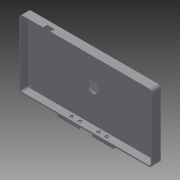
# Autodesk Inventor part: Master Tablet Enclosure
Saved by Autodesk Inventor 2014 SP2 (Build 180246200, 246)
## iProperties
Created: 2015-08-04
Part Number: Master Tablet Enclosure
Material: Generic
Document SubType Name: Modeling
Designer: Devon
Density: 1 g/cm^3
Appearance: Default
Author: Devon
Autodesk Inventor part; units mm, degrees
ref_plane "YZ Plane" through (0, 0, 0) normal (1, 0, 0) x (0, 1, 0)
ref_plane "XZ Plane" through (0, 0, 0) normal (0, 1, 0) x (-1, 0, 0)
sketch "Sketch1" plane through (0, 0, 0) normal (0, 0, 1) x (1, 0, 0)
  line L0 (-10.454202, 14.601943) -> (210.208298, 14.601943)
  line L1 (216.558298, 8.251943) -> (216.558298, -98.110557)
  line L2 (210.208298, -104.460557) -> (-10.454202, -104.460557)
  line L3 (-16.804202, -98.110557) -> (-16.804202, 8.251943)
  line L4 (99.877048, 12.220693) -> (-10.454202, 12.220693)
  line L5 (-14.422952, 8.251943) -> (-14.422952, -44.929307)
  line L6 (99.877048, 12.220693) -> (210.208298, 12.220693)
  line L7 (214.177048, 8.251943) -> (214.177048, -44.929307)
  line L8 (99.877048, -102.079307) -> (210.208298, -102.079307)
  line L9 (214.177048, -98.110557) -> (214.177048, -44.929307)
  line L10 (99.877048, -102.079307) -> (-10.454202, -102.079307)
  line L11 (-14.422952, -98.110557) -> (-14.422952, -44.929307)
  arc A0 (-10.454202, 14.601943) -> (-16.804202, 8.251943) centre (-10.454202, 8.251943) ccw
  arc A1 (216.558298, 8.251943) -> (210.208298, 14.601943) centre (210.208298, 8.251943) ccw
  arc A2 (210.208298, -104.460557) -> (216.558298, -98.110557) centre (210.208298, -98.110557) ccw
  arc A3 (-16.804202, -98.110557) -> (-10.454202, -104.460557) centre (-10.454202, -98.110557) ccw
  arc A4 (-10.454202, 12.220693) -> (-14.422952, 8.251943) centre (-10.454202, 8.251943) ccw
  arc A5 (214.177048, 8.251943) -> (210.208298, 12.220693) centre (210.208298, 8.251943) ccw
  arc A6 (210.208298, -102.079307) -> (214.177048, -98.110557) centre (210.208298, -98.110557) ccw
  arc A7 (-14.422952, -98.110557) -> (-10.454202, -102.079307) centre (-10.454202, -98.110557) ccw
  point P0 (0, 0)
  point P1 (-16.804202, 14.601943)
  point P2 (216.558298, -104.460557)
  point P3 (216.558298, 14.601943)
  point P4 (-16.804202, -104.460557)
  dimension "d0" = 233.3625
  dimension "d1" = 119.0625
  dimension "d9" = 6.35
  dimension "d10" = 3.96875
  constraints: 24 end point, 16 point on circle, 16 tangent, 8 centre point, 8 point on line, 6 equal radius, 4 horizontal, 4 perpendicular, 2 parallel
  measures "d0" distance of point (216.558, -104.461) point (-16.804, -104.461)
  measures "d1" distance of point (216.558, 14.602) point (216.558, -104.461)
  measures "d9" radius of A0
  measures "d10" radius of A4
extrude "Extrusion1" add sketch "Sketch1" along normal blind 2.38125 contours L0 A1 L1 A2 L2 A3 L3 A0 | L6 A5 L7 L9 A6 L8 L10 A7 L11 L5 A4 L4
sketch "Sketch2" plane through (0, 0, 2.38125) normal (0, 0, 1) x (1, 0, 0)
  line L0 (210.208298, 14.601943) -> (-10.454202, 14.601943)
  arc A0 (-10.454202, 14.601943) -> (-16.804202, 8.251943) centre (-10.454202, 8.251943) ccw
  line L1 (-16.804202, 8.251943) -> (-16.804202, -98.110557)
  arc A1 (-16.804202, -98.110557) -> (-10.454202, -104.460557) centre (-10.454202, -98.110557) ccw
  line L2 (-10.454202, -104.460557) -> (210.208298, -104.460557)
  arc A2 (210.208298, -104.460557) -> (216.558298, -98.110557) centre (210.208298, -98.110557) ccw
  line L3 (216.558298, -98.110557) -> (216.558298, 8.251943)
  arc A3 (216.558298, 8.251943) -> (210.208298, 14.601943) centre (210.208298, 8.251943) ccw
  line L4 (99.877048, 12.220693) -> (-10.454202, 12.220693)
  line L5 (-14.422952, 8.251943) -> (-14.422952, -44.929307)
  line L6 (99.877048, -102.079307) -> (-10.454202, -102.079307)
  line L7 (-14.422952, -98.110557) -> (-14.422952, -44.929307)
  line L8 (99.877048, -102.079307) -> (210.208298, -102.079307)
  line L9 (214.177048, -98.110557) -> (214.177048, -44.929307)
  line L10 (99.877048, 12.220693) -> (210.208298, 12.220693)
  line L11 (214.177048, 8.251943) -> (214.177048, -44.929307)
  arc A4 (-10.454202, 12.220693) -> (-14.422952, 8.251943) centre (-10.454202, 8.251943) ccw
  arc A5 (214.177048, 8.251943) -> (210.208298, 12.220693) centre (210.208298, 8.251943) ccw
  arc A6 (210.208298, -102.079307) -> (214.177048, -98.110557) centre (210.208298, -98.110557) ccw
  arc A7 (-14.422952, -98.110557) -> (-10.454202, -102.079307) centre (-10.454202, -98.110557) ccw
  point P0 (0, 0)
  dimension "d15" = 3.96875
  constraints: 16 end point, 8 point on circle, 8 tangent, 4 centre point, 3 equal radius, 2 horizontal, 2 perpendicular
  measures "d15" radius of A4
extrude "Extrusion2" add sketch "Sketch2" along normal blind 2.38125
sketch "Sketch3" plane through (0, 0, 4.7625) normal (0, 0, 1) x (1, 0, 0)
  arc A0 (-10.454202, 12.220693) -> (-14.422952, 8.251943) centre (-10.454202, 8.251943) ccw
  arc A1 (214.177048, 8.251943) -> (210.208298, 12.220693) centre (210.208298, 8.251943) ccw
  line L0 (214.177048, 8.251943) -> (214.177048, -98.110557)
  arc A2 (210.208298, -102.079307) -> (214.177048, -98.110557) centre (210.208298, -98.110557) ccw
  line L1 (210.208298, -102.079307) -> (-10.454202, -102.079307)
  arc A3 (-14.422952, -98.110557) -> (-10.454202, -102.079307) centre (-10.454202, -98.110557) ccw
  line L2 (-14.422952, -98.110557) -> (-14.422952, 8.251943)
  arc A4 (-10.454202, 14.601943) -> (-16.804202, 8.251943) centre (-10.454202, 8.251943) ccw
  line L3 (-16.804202, 8.251943) -> (-16.804202, -98.110557)
  arc A5 (-16.804202, -98.110557) -> (-10.454202, -104.460557) centre (-10.454202, -98.110557) ccw
  line L4 (-10.454202, -104.460557) -> (210.208298, -104.460557)
  arc A6 (210.208298, -104.460557) -> (216.558298, -98.110557) centre (210.208298, -98.110557) ccw
  line L5 (216.558298, -98.110557) -> (216.558298, 8.251943)
  arc A7 (216.558298, 8.251943) -> (210.208298, 14.601943) centre (210.208298, 8.251943) ccw
  line L6 (214.177048, -44.929307) -> (214.177048, -41.754307)
  line L7 (214.177048, -41.754307) -> (216.558298, -41.754307)
  line L8 (216.558298, -41.754307) -> (216.558298, -44.929307)
  line L9 (216.558298, -44.929307) -> (216.558298, -48.104307)
  line L10 (216.558298, -48.104307) -> (214.177048, -48.104307)
  line L11 (214.177048, -48.104307) -> (214.177048, -44.929307)
  line L12 (-14.422952, -44.929307) -> (-14.422952, -41.754307)
  line L13 (-14.422952, -41.754307) -> (-16.804202, -41.754307)
  line L14 (-16.804202, -41.754307) -> (-16.804202, -44.929307)
  line L15 (-16.804202, -44.929307) -> (-16.804202, -48.104307)
  line L16 (-16.804202, -48.104307) -> (-14.422952, -48.104307)
  line L17 (-14.422952, -48.104307) -> (-14.422952, -44.929307)
  line L18 (25.105798, 14.601943) -> (25.105798, 12.220693)
  line L19 (37.805798, 14.601943) -> (37.805798, 12.220693)
  line L20 (-10.454202, 14.601943) -> (25.105798, 14.601943)
  line L21 (25.105798, 12.220693) -> (-10.454202, 12.220693)
  line L22 (37.805798, 12.220693) -> (210.208298, 12.220693)
  line L23 (210.208298, 14.601943) -> (37.805798, 14.601943)
  point P0 (0, 0)
  dimension "d18" = 3.175
  dimension "d19" = 3.175
  dimension "d20" = 3.175
  dimension "d21" = 3.175
  dimension "d78" = 35.56
  dimension "d79" = 12.7
  constraints: 36 end point, 8 point on line, 6 perpendicular, 4 collinear, 4 midpoint, 3 tangent, 1 parallel, 1 point on circle
  measures "d18" distance of L6.start L6.end
  measures "d19" distance of L7.end L8.end
  measures "d20" distance of L8.end L9.end
  measures "d21" distance of L12.start L12.end
  measures "d78" distance of L20.start L18.start
  measures "d79" distance of L18.start L19.start
extrude "Extrusion3" add sketch "Sketch3" along normal blind 10.31875 contours A0 L2 L13 L3 A4 L20 L18 L21 | L2 A3 L1 A2 L0 L10 L5 A6 L4 A5 L3 L16
sketch "Sketch4" plane through (0, 0, 15.08125) normal (0, 0, 1) x (1, 0, 0)
  line L0 (214.177048, -41.754307) -> (216.558298, -41.754307)
  line L1 (216.558298, -41.754307) -> (216.558298, -48.104307)
  line L2 (216.558298, -48.104307) -> (214.177048, -48.104307)
  line L3 (214.177048, -48.104307) -> (214.177048, -41.754307)
  line L4 (-16.804202, -41.754307) -> (-14.422952, -41.754307)
  line L5 (-14.422952, -41.754307) -> (-14.422952, -48.104307)
  line L6 (-14.422952, -48.104307) -> (-16.804202, -48.104307)
  line L7 (-16.804202, -48.104307) -> (-16.804202, -41.754307)
  point P0 (0, 0)
  dimension "d24" = 2.38125
  dimension "d25" = 6.35
  dimension "d26" = 2.38125
  dimension "d27" = 6.35
  constraints: 16 end point, 4 parallel, 2 horizontal, 2 perpendicular
  measures "d24" distance of L1.end L2.end
  measures "d25" distance of L0.end L1.end
  measures "d26" distance of L5.end L6.end
  measures "d27" distance of L4.end L5.end
extrude "Extrusion4" add sketch "Sketch4" against normal blind 7.9375
sketch "Sketch5" plane through (0, 0, 0) normal (0, 0, -1) x (-1, 0, 0)
  arc A0 (-210.208298, 14.601943) -> (-216.558298, 8.251943) centre (-210.208298, 8.251943) ccw
  line L0 (-210.208298, 8.251943) -> (-99.877048, 8.251943)
  line L1 (-99.877048, 8.251943) -> (-99.877048, -44.929307)
  line L2 (-99.877048, -44.929307) -> (-210.208298, -44.929307)
  line L3 (-210.208298, -44.929307) -> (-210.208298, 8.251943)
  point P0 (0, 0)
  constraints: 8 end point, 2 parallel, 1 horizontal, 1 perpendicular
hole "Hole1" at (99.877048, -44.929307, 0) direction (0, 0, 1) diameter 19.05 end through all
sketch "Sketch7" plane through (-10.454202, -104.460557, 0) normal (0, -1, 0) x (1, 0, 0)
  line L0 (220.6625, 0) -> (0, 0)
  line L1 (0, 15.08125) -> (220.6625, 15.08125)
  line L2 (61.11875, 15.08125) -> (61.11875, 0)
  line L3 (159.54375, 15.08125) -> (159.54375, 0)
  line L4 (61.11875, 15.08125) -> (159.54375, 15.08125)
  line L5 (159.54375, 0) -> (61.11875, 0)
  point P0 (10.454202, 0)
  constraints: 8 end point, 4 point on line, 2 perpendicular, 1 collinear, 1 parallel
extrude "Extrusion5" add sketch "Sketch7" along normal blind 25.4
sketch "Sketch8" plane through (149.089548, -104.460557, 15.08125) normal (1, 0, 0) x (0, 0, -1)
  line L0 (15.08125, 0) -> (-19.502452, -9.266675)
  line L1 (15.08125, 0) -> (50.884933, 0) construction
  point P0 (15.08125, 104.460557)
  dimension "d41" = 165
  constraints: 4 end point, 1 equal length, 1 horizontal
  measures "d41" angle of L0 L1
split body "Split1" sketch "Sketch8" result one side removed curves L0 removed pieces at (116.281215, -121.39389, 0.5)
ref_plane "Work Plane1" through (50.664548, -102.160446, 0.616313) normal (0, -0.9659258, -0.258819) x (1, 0, 0)
sketch "Sketch10" plane through (0, 0, 15.08125) normal (0, 0, 1) x (1, 0, 0)
  line L0 (99.877048, -104.460557) -> (111.307048, -104.460557)
  line L1 (111.307048, -104.460557) -> (111.307048, -108.501565)
  line L2 (99.877048, -104.460557) -> (88.447048, -104.460557)
  line L3 (88.447048, -104.460557) -> (88.447048, -108.501565)
  line L4 (88.447048, -108.501565) -> (111.307048, -108.501565)
  point P0 (0, 0)
  dimension "d43" = 11.43
  dimension "d44" = 11.43
  constraints: 10 end point, 1 perpendicular
  measures "d43" distance of L0.start L0.end
  measures "d44" distance of L0.start L2.end
split body "Split2" sketch "Sketch10" result one side removed curves L4 L1 L0 L2 L3 removed pieces at (99.877048, -106.671599, 10.183576)
sketch "Sketch13" plane through (50.664548, -102.160446, 0.616313) normal (0, -0.9659258, -0.258819) x (1, 0, 0)
  line L0 (37.7825, 0) -> (37.7825, 15.613259)
  line L1 (0, 15.613259) -> (37.7825, 15.613259)
  line L2 (0, 0) -> (0, 15.613259)
  line L3 (37.7825, 0) -> (0, 0)
  line L4 (60.6425, 15.613259) -> (60.6425, 0)
  line L5 (98.425, 0) -> (60.6425, 0)
  line L6 (98.425, 15.613259) -> (98.425, 0)
  line L7 (60.6425, 15.613259) -> (98.425, 15.613259)
  line L8 (0, 15.613259) -> (98.425, 15.613259)
  line L9 (49.2125, 15.613259) -> (49.2125, 0)
  line L10 (49.2125, 7.806629) -> (32.8295, 7.806629)
  line L11 (49.2125, 7.806629) -> (65.5955, 7.806629)
  line L12 (65.5955, 7.806629) -> (80.0735, 7.806629)
  line L13 (32.8295, 7.806629) -> (18.3515, 7.806629)
  point P0 (-50.664548, -27.036381)
  dimension "d45" = 16.383
  dimension "d46" = 16.383
  dimension "d47" = 14.478
  dimension "d48" = 14.478
  constraints: 12 end point, 4 collinear, 2 midpoint, 2 perpendicular
  measures "d45" distance of L10.start L10.end
  measures "d46" distance of L10.start L11.end
  measures "d47" distance of L11.end L12.end
  measures "d48" distance of L10.end L13.end
hole "Hole2" at (69.016048, -104.18095, 8.156938) at (116.260048, -104.18095, 8.156938) at (83.494048, -104.18095, 8.156938) at (130.738048, -104.18095, 8.156938) direction (0, 0.9659258, 0.258819) diameter 6.35 end through all
sketch "Sketch14" plane through (50.664548, -102.160446, 0.616313) normal (0, -0.9659258, -0.258819) x (1, 0, 0)
  line L0 (37.7825, 0) -> (37.7825, 15.613259)
  line L1 (0, 15.613259) -> (37.7825, 15.613259)
  line L2 (0, 0) -> (0, 15.613259)
  line L3 (37.7825, 0) -> (0, 0)
  line L4 (60.6425, 15.613259) -> (60.6425, 0)
  line L5 (98.425, 0) -> (60.6425, 0)
  line L6 (98.425, 15.613259) -> (98.425, 0)
  line L7 (60.6425, 15.613259) -> (98.425, 15.613259)
  line L8 (0, 15.613259) -> (98.425, 15.613259)
  line L9 (49.2125, 15.613259) -> (49.2125, 0)
  line L10 (49.2125, 7.806629) -> (65.5955, 7.806629)
  line L11 (65.5955, 7.806629) -> (80.0735, 7.806629)
  line L12 (49.2125, 7.806629) -> (32.8295, 7.806629)
  line L13 (32.8295, 7.806629) -> (18.3515, 7.806629)
  point P0 (-50.664548, -27.036381)
  dimension "d56" = 16.383
  dimension "d57" = 14.478
  dimension "d58" = 16.383
  dimension "d59" = 14.478
  constraints: 12 end point, 3 collinear, 2 midpoint, 2 perpendicular, 1 parallel
  measures "d56" distance of L10.start L10.end
  measures "d57" distance of L10.end L11.end
  measures "d58" distance of L10.start L12.end
  measures "d59" distance of L12.end L13.end
hole "Hole3" at (69.016048, -104.18095, 8.156938) at (83.494048, -104.18095, 8.156938) at (116.260048, -104.18095, 8.156938) at (130.738048, -104.18095, 8.156938) direction (0, -0.9659258, -0.258819) diameter 3.175 end through all
sketch "Sketch15" plane through (0, 0, 4.7625) normal (0, 0, 1) x (1, 0, 0)
  line L0 (216.558298, -41.754307) -> (214.177048, -41.754307)
  line L1 (214.177048, 8.251943) -> (214.177048, -48.104307)
  line L2 (216.558298, -41.754307) -> (214.177048, -41.754307)
  line L3 (214.177048, -41.754307) -> (214.177048, -48.104307)
  line L4 (214.177048, -48.104307) -> (216.558298, -48.104307)
  line L5 (216.558298, -48.104307) -> (216.558298, -41.754307)
  point P0 (0, 0)
  constraints: 8 end point, 2 parallel, 1 horizontal, 1 perpendicular
extrude "Extrusion6" add sketch "Sketch15" along normal blind 2.3876
sketch "Sketch16" plane through (0, 0, 4.7625) normal (0, 0, 1) x (1, 0, 0)
  line L0 (-14.422952, -41.754307) -> (-16.804202, -41.754307)
  line L1 (-16.804202, -41.754307) -> (-16.804202, -48.104307)
  line L2 (-14.422952, -41.754307) -> (-16.804202, -41.754307)
  line L3 (-16.804202, -41.754307) -> (-16.804202, -48.104307)
  line L4 (-16.804202, -48.104307) -> (-14.422952, -48.104307)
  line L5 (-14.422952, -48.104307) -> (-14.422952, -41.754307)
  point P0 (0, 0)
  constraints: 8 end point, 2 parallel, 1 horizontal, 1 perpendicular
extrude "Extrusion7" add sketch "Sketch16" along normal blind 2.3876
sketch "Sketch17" plane through (0, 0, 0) normal (0, 0, -1) x (-1, 0, 0)
  arc A0 (10.454202, -104.460557) -> (16.804202, -98.110557) centre (10.454202, -98.110557) ccw
  arc A1 (16.804202, 8.251943) -> (10.454202, 14.601943) centre (10.454202, 8.251943) ccw
  arc A2 (-210.208298, 14.601943) -> (-216.558298, 8.251943) centre (-210.208298, 8.251943) ccw
  arc A3 (-216.558298, -98.110557) -> (-210.208298, -104.460557) centre (-210.208298, -98.110557) ccw
  point P0 (0, 0)
hole "Hole4" at (210.208298, 8.251943, 0) at (-10.454202, 8.251943, 0) at (-10.454202, -98.110557, 0) at (210.208298, -98.110557, 0) direction (0, 0, 1) diameter 3.175 end through all
sketch "Sketch18" plane through (0, 0, 4.7625) normal (0, 0, 1) x (1, 0, 0)
  line L0 (214.177048, -41.754307) -> (216.558298, -41.754307)
  line L1 (216.558298, -41.754307) -> (216.558298, 8.251943)
  arc A0 (216.558298, 8.251943) -> (210.208298, 14.601943) centre (210.208298, 8.251943) ccw
  line L2 (210.208298, 14.601943) -> (25.105798, 14.601943)
  line L3 (25.105798, 12.220693) -> (210.208298, 12.220693)
  arc A1 (214.177048, 8.251943) -> (210.208298, 12.220693) centre (210.208298, 8.251943) ccw
  line L4 (214.177048, 8.251943) -> (214.177048, -41.754307)
  line L5 (25.105798, 14.601943) -> (37.805798, 14.601943)
  line L6 (37.805798, 14.601943) -> (37.805798, 12.220693)
  point P0 (0, 0)
  dimension "d80" = 12.7
  constraints: 4 end point, 2 point on line, 1 perpendicular
  measures "d80" distance of L2.end L5.end
extrude "Extrusion8" add sketch "Sketch18" along normal blind 10.3124
sketch "Sketch19" plane through (0, 0, 4.7625) normal (0, 0, 1) x (1, 0, 0)
  line L0 (37.805798, 12.220693) -> (37.805798, 14.601943)
  line L1 (37.805798, 14.601943) -> (25.105798, 14.601943)
  line L2 (25.105798, 14.601943) -> (25.105798, 12.220693)
  line L3 (25.105798, 12.220693) -> (37.805798, 12.220693)
  point P0 (0, 0)
extrude "Extrusion9" add sketch "Sketch19" along normal blind 2.6924
body "Solid1"
